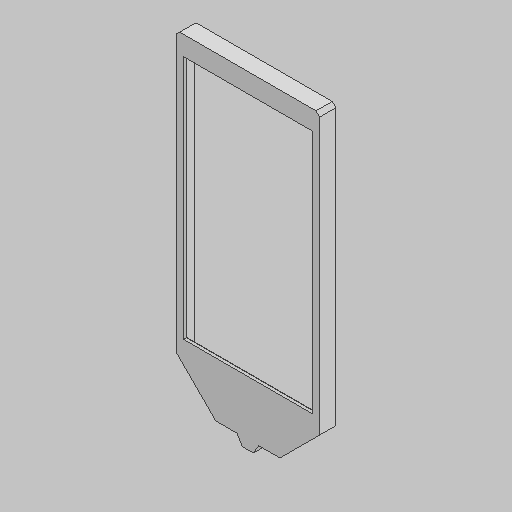
# Autodesk Inventor part: BiselTelefono
Saved by Autodesk Inventor 2025.3 (Build 293356000, 356)
## iProperties
Created: 2025-11-09
Part Number: BiselTelefono
Material: Genérico
Document SubType Name: Modeling
Designer: Inema
Density: 1 g/cm^3
Appearance: Valor por defecto
Author: Inema
Autodesk Inventor part; units mm, degrees
ref_plane "YZ Plane" through (0, 0, 0) normal (1, 0, 0) x (0, 1, 0)
ref_plane "XZ Plane" through (0, 0, 0) normal (0, 1, 0) x (-1, 0, 0)
ref_plane "XY Plane" through (0, 0, 0) normal (0, 0, 1) x (1, 0, 0)
sketch "Boceto1" plane through (0, 0, 0) normal (0, 0, 1) x (1, 0, 0)
  line L0 (-39.75, -78.25) -> (39.75, -78.25)
  line L1 (39.75, -78.25) -> (39.75, 78.25)
  line L2 (39.75, 78.25) -> (-39.75, 78.25)
  line L3 (-39.75, 78.25) -> (-39.75, -78.25)
  line L4 (-39.75, -78.25) -> (39.75, 78.25) construction
  line L5 (39.75, -78.25) -> (-39.75, 78.25) construction
  point P0 (0, 0)
  dimension "d0" = 79.5
  dimension "d1" = 156.5
  constraints: 12 end point, 2 midpoint, 2 parallel, 1 horizontal, 1 perpendicular
  measures "d0" distance of L0.start L0.end
  measures "d1" distance of L0.end L1.end
extrude "Extrusión1" add sketch "Boceto1" along normal blind 9
sketch "Boceto2" plane through (0, 0, 9) normal (0, 0, 1) x (1, 0, 0)
  line L0 (-39.75, -78.25) -> (39.75, -78.25) projected
  line L1 (-6, -78.25) -> (-6, -98.25)
  line L2 (-6, -98.25) -> (-3, -103.25)
  line L3 (-3, -103.25) -> (3, -103.25)
  line L4 (3, -103.25) -> (6, -98.25)
  line L5 (6, -98.25) -> (6, -78.25)
  point P0 (0, 0)
  point P1 (6, -88.25)
  point P2 (-6, -88.25)
  point P3 (0, -78.25)
  point P4 (0, -103.25)
  point P5 (0, -78.25)
  dimension "d4" = 12
  dimension "d5" = 6
  dimension "d6" = 20
  dimension "d7" = 5
  dimension "d8" = 6
  constraints: 10 end point, 5 midpoint, 2 parallel, 2 point on line, 1 perpendicular, 1 vertical, 1 vertical alignment
  measures "d4" distance of point (6, -88.25) point (-6, -88.25)
  measures "d5" distance from line of L5 point (0, -78.25)
  measures "d6" distance of L4.end L5.end
  measures "d7" vertical distance of L3.end L4.end
  measures "d8" distance of L2.end L3.end
extrude "Extrusión2" add sketch "Boceto2" against normal up to surface (9 mm away)
chamfer "Chaflán2" distance 2 angle 45 4 edges at (-39.75, -78.25, 4.5) (-39.75, 78.25, 4.5) (39.75, -78.25, 4.5) (39.75, 78.25, 4.5)
shell "Vaciado1" thickness 1 removed faces 2 at (-2, 24.75, 0) at (-1, -103.25, 6)
sketch "Boceto3" plane through (0, 0, 9) normal (0, 0, 1) x (1, 0, 0)
  line L0 (-34.75, 66.75) -> (34.75, 66.75)
  line L1 (34.75, 66.75) -> (34.75, -67.25)
  line L2 (34.75, -67.25) -> (-34.75, -67.25)
  line L3 (-34.75, -67.25) -> (-34.75, 66.75)
  line L4 (-34.75, 66.75) -> (34.75, -67.25) construction
  line L5 (34.75, 66.75) -> (-34.75, -67.25) construction
  line L6 (37.3358, 77.25) -> (38.75, 75.8358) projected
  line L7 (38.75, -75.8358) -> (38.75, 75.8358) projected
  line L8 (38.75, -75.8358) -> (37.3358, -77.25) projected
  line L9 (5, -77.25) -> (37.3358, -77.25) projected
  line L10 (5, -97.973) -> (5, -77.25) projected
  line L11 (1.8338, -103.25) -> (5, -97.973) projected
  line L12 (-1.8338, -103.25) -> (1.8338, -103.25) projected
  line L13 (-5, -97.973) -> (-1.8338, -103.25) projected
  line L14 (-5, -77.25) -> (-5, -97.973) projected
  line L15 (-37.3358, -77.25) -> (-5, -77.25) projected
  line L16 (-37.3358, -77.25) -> (-38.75, -75.8358) projected
  line L17 (-38.75, 75.8358) -> (-38.75, -75.8358) projected
  line L18 (-38.75, 75.8358) -> (-37.3358, 77.25) projected
  line L19 (37.3358, 77.25) -> (-37.3358, 77.25) projected
  point P0 (0, 0)
  point P1 (0, -0.25)
  dimension "d18" = 4
  dimension "d19" = 4
  dimension "d20" = 10.5
  dimension "d21" = 10
  constraints: 12 end point, 2 midpoint, 2 parallel, 1 horizontal, 1 perpendicular
  measures "d18" distance between parallel lines of L3 L17
  measures "d19" distance between parallel lines of L1 L7
  measures "d20" distance between parallel lines of L0 L19
  measures "d21" distance between parallel lines of L2 L9
extrude "Extrusión3" cut sketch "Boceto3" against normal blind 10 contours L0 L1 L2 L3
chamfer "Chaflán3" distance 0.8 angle 45 4 edges at (0, 66.75, 9) (34.75, -0.25, 9) (0, -67.25, 9) (-34.75, -0.25, 9)
move faces "Desplazar1" translate (0, -20, 0) faces at (-27.1667, -78.25, 3) (16.5833, -78.25, 3) (-26.5572, -77.25, 2.6667) (26.5572, -77.25, 5.3333)
equation "\"d5\" = 0.5 * d4"
